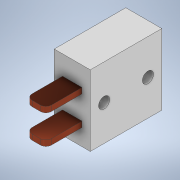
# Autodesk Inventor part: Switch
Saved by Autodesk Inventor 2020 (Build 240168000, 168)
## iProperties
Created: 2023-12-15
Part Number: Switch
Material: Generic
Document SubType Name: Modeling
Designer: smz3rm
Density: 2.00394 g/cm^3
Appearance: Default
Mass: 2.15 g
Surface Area: 8.45081 cm^2
Volume: 1.07289 cm^3
Author: smz3rm
Autodesk Inventor part; units mm, degrees
ref_plane "YZ Plane" through (0, 0, 0) normal (1, 0, 0) x (0, 1, 0)
ref_plane "XZ Plane" through (0, 0, 0) normal (0, 1, 0) x (-1, 0, 0)
ref_plane "XY Plane" through (0, 0, 0) normal (0, 0, 1) x (1, 0, 0)
sketch "Sketch1" plane through (0, 0, 0) normal (1, 0, 0) x (0, 1, 0)
  line L0 (6.375, 6.45) -> (-6.375, 6.45)
  line L1 (-6.375, 6.45) -> (-6.375, -6.45)
  line L2 (-6.375, -6.45) -> (6.375, -6.45)
  line L3 (6.375, -6.45) -> (6.375, 6.45)
  line L4 (6.375, 6.45) -> (-6.375, -6.45) construction
  line L5 (-6.375, 6.45) -> (6.375, -6.45) construction
  circle A0 centre (0, -3.95) radius 1
  circle A1 centre (0, 3.95) radius 1
  line L6 (0, 6.45) -> (0, -6.45)
  point P0 (0, 0)
  dimension "d0" = 12.75
  dimension "d1" = 12.9
  dimension "d2" = 2
  dimension "d3" = 2.5
  dimension "d4" = 2
  dimension "d5" = 2.5
  constraints: 14 end point, 4 midpoint, 2 centre point, 2 parallel, 2 point on line, 1 horizontal, 1 perpendicular
  measures "d0" distance of L2.end L1.end
  measures "d1" distance of L0.end L1.end
  measures "d2" diameter of A0
  measures "d3" distance from line of L2 A0.centre
  measures "d4" diameter of A1
  measures "d5" distance from line of L0 A1.centre
extrude "Extrusion1" add sketch "Sketch1" along normal blind 6.5 contours L3 L2 L6 A0 A1 L0 | L6 A1 A0 L2 L1 L0
sketch "Sketch2" plane through (0, -6.375, 6.45) normal (0, 0, 1) x (1, 0, 0)
  line L0 (1.5, 9.25) -> (5, 9.25)
  line L1 (5, 9.25) -> (5, 8.25)
  line L2 (5, 8.25) -> (1.5, 8.25)
  line L3 (1.5, 8.25) -> (1.5, 9.25)
  line L4 (1.5, 9.25) -> (5, 8.25) construction
  line L5 (5, 9.25) -> (1.5, 8.25) construction
  line L6 (1.5, 4) -> (5, 4)
  line L7 (5, 4) -> (5, 3)
  line L8 (5, 3) -> (1.5, 3)
  line L9 (1.5, 3) -> (1.5, 4)
  line L10 (1.5, 4) -> (5, 3) construction
  line L11 (5, 4) -> (1.5, 3) construction
  line L12 (0, 12.75) -> (6.5, 12.75) projected
  line L13 (3.25, 12.75) -> (3.25, 0)
  line L14 (0, 0) -> (6.5, 0) projected
  point P0 (0, 6.375)
  point P1 (3.25, 8.75)
  point P2 (3.25, 3.5)
  point P3 (3.25, 8.75)
  point P4 (3.25, 3.5)
  dimension "d8" = 3.5
  dimension "d9" = 1
  dimension "d12" = 3.5
  dimension "d13" = 3.5
  constraints: 26 end point, 8 midpoint, 4 parallel, 2 equal length, 2 horizontal, 2 perpendicular, 2 point on line, 1 vertical
  measures "d8" distance of L1.end L2.end
  measures "d9" distance of L0.end L1.end
  measures "d12" distance between parallel lines of L12 L0
  measures "d13" distance from line of L14 point (3.25, 3.5)
extrude "Extrusion2" add sketch "Sketch2" along normal blind 6.5
fillet "Fillet1" radius 1 4 edges at (5, 2.375, 12.95) (1.5, 2.375, 12.95) (1.5, -2.875, 12.95) (5, -2.875, 12.95)
equation "\"d13\" = d12"
body "Solid1"
